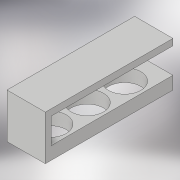
# Autodesk Inventor part: piston align
Saved by Autodesk Inventor 2019 (Build 230136000, 136)
## iProperties
Created: 2020-06-05
Part Number: piston align
Material: Generic
Document SubType Name: Modeling
Designer: Manoj
Density: 1 g/cm^3
Appearance: Default
Author: Manoj
Autodesk Inventor part; units mm, degrees
ref_plane "YZ Plane" through (0, 0, 0) normal (1, 0, 0) x (0, 1, 0)
ref_plane "XZ Plane" through (0, 0, 0) normal (0, 1, 0) x (-1, 0, 0)
ref_plane "XY Plane" through (0, 0, 0) normal (0, 0, 1) x (1, 0, 0)
sketch "Sketch2" plane through (0, 0, 0) normal (0, 1, 0) x (-1, 0, 0)
  line L0 (0, 0) -> (150, 0)
  line L1 (150, 0) -> (150, -500)
  line L2 (150, -500) -> (0, -500)
  line L3 (0, -500) -> (0, 0)
  line L4 (75, 0) -> (75, -93.5) construction
  circle A0 centre (75, -93.5) radius 63.5
  circle A1 centre (75, -239.702) radius 63.5
  circle A2 centre (75, -385.904) radius 63.5
  dimension "d9" = 150
  dimension "d10" = 500
  dimension "d11" = 93.5
  dimension "d12" = 127
  dimension "d13" = 127
  dimension "d14" = 127
  dimension "d15" = 146.202
  dimension "d16" = 146.202
  constraints: 10 end point, 3 centre point, 2 parallel, 1 coincident, 1 horizontal, 1 midpoint, 1 perpendicular, 1 vertical
  measures "d9" distance of L1.end L2.end
  measures "d10" distance of L0.end L1.end
  measures "d11" distance of L4.start L4.end
  measures "d12" diameter of A0
  measures "d13" diameter of A1
  measures "d14" diameter of A2
  measures "d15" distance of A1.centre L4.end
  measures "d16" distance of A2.centre A1.centre
extrude "Extrusion1" add sketch "Sketch2" along normal blind 50
sketch "Sketch3" plane through (0, 50, 0) normal (0, 1, 0) x (1, 0, 0)
  line L0 (-150, 500) -> (-150, 0) projected
  line L1 (-150, 0) -> (0, 0) projected
  line L2 (-150, 0) -> (0, 0)
  line L3 (0, 0) -> (0, 22.5702)
  line L4 (0, 0) -> (0, 500) projected
  line L5 (-150, 22.5702) -> (-150, 0)
  line L6 (-150, 22.5702) -> (0, 22.5702)
  constraints: 8 end point, 2 equal length, 1 horizontal, 1 point on line
extrude "Extrusion2" add sketch "Sketch3" along normal blind 100
sketch "Sketch4" plane through (0, 150, 0) normal (0, 1, 0) x (1, 0, 0)
  line L0 (0, 0) -> (-150, 0) projected
  line L1 (0, 500) -> (0, 0) projected
  line L2 (-150, 0) -> (0, 0)
  line L3 (0, 0) -> (0, 500)
  line L4 (0, 500) -> (-150, 500)
  line L5 (-150, 500) -> (-150, 0)
  constraints: 8 end point, 2 parallel, 1 horizontal, 1 perpendicular
extrude "Extrusion3" add sketch "Sketch4" along normal blind 25
body "Solid1"
